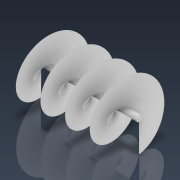
# Autodesk Inventor part: Screw shaft
Saved by Autodesk Inventor 2021.1 (Build 251245010, 245A)
## iProperties
Created: 2021-01-03
Part Number: Screw shaft
Material: 一般
Document SubType Name: Modeling
Designer: User
Density: 1 g/cm^3
Appearance: 預設
Author: User
Autodesk Inventor part; units mm, degrees
ref_plane "YZ Plane" through (0, 0, 0) normal (1, 0, 0) x (0, 1, 0)
ref_plane "XZ Plane" through (0, 0, 0) normal (0, 1, 0) x (-1, 0, 0)
ref_plane "XY Plane" through (0, 0, 0) normal (0, 0, 1) x (1, 0, 0)
sketch "草圖1" plane through (0, 0, 0) normal (0, 0, 1) x (1, 0, 0)
  line L0 (-348.7345, 0) -> (348.7345, 0)
  line L1 (348.7345, 0) -> (348.7345, -20)
  line L2 (348.7345, -20) -> (-348.7345, -20)
  line L3 (-348.7345, -20) -> (-348.7345, 0)
  line L4 (-348.7345, 0) -> (-358.7345, 0)
  line L5 (-358.7345, 0) -> (-358.7345, -10)
  line L6 (-358.7345, -10) -> (-348.7345, -10)
  line L7 (-348.7345, -10) -> (-348.7345, 0)
  line L8 (348.7345, 0) -> (358.7345, 0)
  line L9 (358.7345, 0) -> (358.7345, -10)
  line L10 (358.7345, -10) -> (348.7345, -10)
  line L11 (348.7345, -10) -> (348.7345, 0)
  point P0 (0, 0)
  point P1 (0, 0)
  dimension "d0" = 697.469
  dimension "d1" = 40
  dimension "d2" = 20
  dimension "d3" = 10
  dimension "d4" = 20
  dimension "d5" = 10
  constraints: 24 end point, 6 parallel, 3 horizontal, 3 perpendicular, 1 coincident, 1 midpoint
  measures "d0" distance of L1.end L2.end
  measures "d1" diameter of L2 L0
  measures "d2" diameter of L6 L4
  measures "d3" distance of L5.end L6.end
  measures "d4" diameter of L10 L8
  measures "d5" distance of L9.end L10.end
revolve "迴轉1" add sketch "草圖1" angle 360 about axis through (-348.7345, 0, 0) along (1, 0, 0)
sketch "草圖2" plane through (0, 0, 0) normal (0, 0, 1) x (1, 0, 0)
  line L0 (358.7345, 10) -> (358.7345, -10) construction
  line L1 (358.7345, -10) -> (348.7345, -10) construction
  line L2 (348.7345, -10) -> (348.7345, -20) construction
  line L3 (348.7345, -20) -> (-348.7345, -20) construction
  line L4 (-348.7345, -20) -> (-348.7345, -10) construction
  line L5 (-348.7345, -10) -> (-358.7345, -10) construction
  line L6 (-358.7345, -10) -> (-358.7345, 10) construction
  line L7 (-358.7345, 10) -> (-348.7345, 10) construction
  line L8 (-348.7345, 10) -> (-348.7345, 20) construction
  line L9 (-348.7345, 20) -> (348.7345, 20) construction
  line L10 (348.7345, 20) -> (348.7345, 10) construction
  line L11 (348.7345, 10) -> (358.7345, 10) construction
  line L12 (348.7345, -20) -> (348.7345, -342.9396) construction
  line L13 (346.2345, -215) -> (348.7345, -215)
  line L14 (348.7345, -215) -> (348.7345, -20)
  line L15 (348.7345, -20) -> (346.2345, -20)
  line L16 (346.2345, -20) -> (346.2345, -215)
  line L17 (358.7345, -10) -> (348.7345, -10) construction
  line L18 (348.7345, -10) -> (348.7345, -20) construction
  line L19 (348.7345, -20) -> (-348.7345, -20) construction
  line L20 (-348.7345, -20) -> (-348.7345, -10) construction
  line L21 (-348.7345, -10) -> (-358.7345, -10) construction
  line L22 (-358.7345, 10) -> (-348.7345, 10) construction
  line L23 (-348.7345, 10) -> (-348.7345, 20) construction
  line L24 (-348.7345, 20) -> (348.7345, 20) construction
  line L25 (348.7345, 20) -> (348.7345, 10) construction
  line L26 (348.7345, 10) -> (358.7345, 10) construction
  line L27 (358.7345, 10) -> (358.7345, -10) projected
  line L28 (-358.7345, -10) -> (-358.7345, 10) projected
  point P0 (0, 0)
  dimension "d9" = 2.5
  dimension "d10" = 215
  constraints: 10 end point, 2 collinear, 2 parallel, 1 horizontal, 1 perpendicular, 1 vertical
  measures "d9" distance of L13.start L13.end
  measures "d10" distance from line of L13 point (0, 0)
coil "螺旋1" sketch "草圖2" operation add axis through (-10, 0, 0) along (-1, 0, 0) pitch 173.5 turns 4 hand left
equation "\"d4\" = d2"
equation "\"d5\" = d3"
